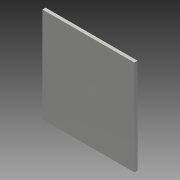
# Autodesk Inventor part: Solar Panel PCB
Saved by Autodesk Inventor 2015 SP1 (Build 190203100, 203)
## iProperties
Created: 2015-06-25
Part Number: Solar Panel PCB
Material: Generic
Document SubType Name: Modeling
Designer: Kartikye
Density: 1 g/cm^3
Appearance: Default
Author: Kartikye
Autodesk Inventor part; units mm, degrees
ref_plane "YZ Plane" through (0, 0, 0) normal (1, 0, 0) x (0, 1, 0)
ref_plane "XZ Plane" through (0, 0, 0) normal (0, 1, 0) x (-1, 0, 0)
ref_plane "XY Plane" through (0, 0, 0) normal (0, 0, 1) x (1, 0, 0)
sketch "Sketch1" plane through (0, 0, 0) normal (0, 1, 0) x (-1, 0, 0)
  line L0 (-23.4, 24.2) -> (23.4, 24.2)
  line L1 (23.4, 24.2) -> (23.4, -24.2)
  line L2 (23.4, -24.2) -> (-23.4, -24.2)
  line L3 (-23.4, -24.2) -> (-23.4, 24.2)
  line L4 (-23.4, 24.2) -> (23.4, -24.2) construction
  line L5 (23.4, 24.2) -> (-23.4, -24.2) construction
  point P0 (0, 0)
  dimension "d0" = 46.8
  dimension "d1" = 48.4
  constraints: 12 end point, 2 midpoint, 2 parallel, 1 horizontal, 1 perpendicular
  measures "d0" distance of L1.end L2.end
  measures "d1" distance of L0.end L1.end
extrude "Extrusion1" add sketch "Sketch1" along normal blind 1.6
body "Solid1"
